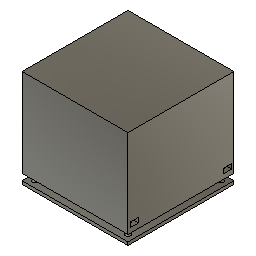
Indoors Test Enclosure (Autodesk Fusion 360 design; units mm, degrees)
Autodesk Fusion 360 part; units mm, degrees
note: some values were not read from the file. Set by a fixed rule: which sketch regions a step uses.
sketch "Sketch1" plane through (0, 0, 0) normal (0, 0, 1) x (1, 0, 0)
  line L0 (25.5, 25.5) -> (-25.5, 25.5)
  line L1 (-25.5, 25.5) -> (-25.5, -25.5)
  line L2 (-25.5, -25.5) -> (25.5, -25.5)
  line L3 (25.5, -25.5) -> (25.5, 25.5)
  line L4 (25.5, 25.5) -> (-25.5, -25.5) construction
  line L5 (-25.5, 25.5) -> (25.5, -25.5) construction
  circle A0 centre (0, 0) radius 22.6
  line L6 (-33, 33) -> (33, 33)
  line L7 (33, 33) -> (33, -33)
  line L8 (33, -33) -> (-33, -33)
  line L9 (-33, -33) -> (-33, 33)
  line L10 (-33, 33) -> (33, -33) construction
  line L11 (33, 33) -> (-33, -33) construction
  circle A1 centre (-29, 29) radius 1.6
  circle A2 centre (29, 29) radius 1.6
  circle A3 centre (-29, -29) radius 1.6
  circle A4 centre (29, -29) radius 1.6
  line L12 (-12.5, -12.5) -> (12.5, -12.5)
  line L13 (12.5, -12.5) -> (12.5, 12.5)
  line L14 (12.5, 12.5) -> (-12.5, 12.5)
  line L15 (-12.5, 12.5) -> (-12.5, -12.5)
  line L16 (-12.5, -12.5) -> (12.5, 12.5) construction
  line L17 (12.5, -12.5) -> (-12.5, 12.5) construction
  line L18 (-26, 29) -> (-27.5, 31.5981)
  line L19 (-27.5, 31.5981) -> (-30.5, 31.5981)
  line L20 (-30.5, 31.5981) -> (-32, 29)
  line L21 (-32, 29) -> (-30.5, 26.4019)
  line L22 (-30.5, 26.4019) -> (-27.5, 26.4019)
  line L23 (-27.5, 26.4019) -> (-26, 29)
  line L24 (30.5, 31.5981) -> (27.5, 31.5981)
  line L25 (32, 29) -> (30.5, 31.5981)
  line L26 (30.5, 26.4019) -> (32, 29)
  line L27 (27.5, 26.4019) -> (30.5, 26.4019)
  line L28 (26, 29) -> (27.5, 26.4019)
  line L29 (27.5, 31.5981) -> (26, 29)
  line L30 (-27.5, -26.4019) -> (-30.5, -26.4019)
  line L31 (-26, -29) -> (-27.5, -26.4019)
  line L32 (-27.5, -31.5981) -> (-26, -29)
  line L33 (-30.5, -31.5981) -> (-27.5, -31.5981)
  line L34 (-32, -29) -> (-30.5, -31.5981)
  line L35 (-30.5, -26.4019) -> (-32, -29)
  line L36 (30.5, -26.4019) -> (27.5, -26.4019)
  line L37 (32, -29) -> (30.5, -26.4019)
  line L38 (30.5, -31.5981) -> (32, -29)
  line L39 (27.5, -31.5981) -> (30.5, -31.5981)
  line L40 (26, -29) -> (27.5, -31.5981)
  line L41 (27.5, -26.4019) -> (26, -29)
  line L42 (-27.5, 31.5981) -> (-36.4083, 31.5981)
  line L43 (-36.4083, 31.5981) -> (-36.4083, 26.4019)
  line L44 (-36.4083, 26.4019) -> (-27.5, 26.4019)
  line L45 (-27.5, 26.4019) -> (-27.5, 31.5981)
  line L46 (-27.5, -26.4019) -> (-35.7888, -26.4019)
  line L47 (-35.7888, -26.4019) -> (-35.7888, -31.5981)
  line L48 (-35.7888, -31.5981) -> (-27.5, -31.5981)
  line L49 (-27.5, -31.5981) -> (-27.5, -26.4019)
  line L50 (27.5, 31.5981) -> (36.8588, 31.5981)
  line L51 (36.8588, 31.5981) -> (36.8588, 26.4019)
  line L52 (36.8588, 26.4019) -> (27.5, 26.4019)
  line L53 (27.5, 26.4019) -> (27.5, 31.5981)
  line L54 (27.5, -26.4019) -> (36.5392, -26.4019)
  line L55 (36.5392, -26.4019) -> (36.5392, -31.5981)
  line L56 (36.5392, -31.5981) -> (27.5, -31.5981)
  line L57 (27.5, -31.5981) -> (27.5, -26.4019)
  point P0 (29, 29)
  point P1 (-29, -29)
  point P2 (29, -29)
  point P3 (-29, 29)
  dimension "d1" = 51
  dimension "d2" = 51
  dimension "d3" = 45.2
  dimension "d4" = 66
  dimension "d5" = 66
  dimension "d6" = 3.2
  dimension "d9" = 58
  dimension "d10" = -58
  dimension "d13" = 58
  dimension "d14" = -58
  dimension "d23" = 25
  dimension "d24" = 25
  dimension "d28" = 3
  dimension "d31" = 58
  dimension "d32" = -58
  constraint horizontal L0
  constraint perpendicular L0 L1
  constraint parallel L0 L2
  constraint parallel L1 L3
  constraint coincident L4 A0.centre
  constraint coincident L5 A0.centre
  constraint coincident A0.centre origin
  constraint horizontal L6
  constraint perpendicular L6 L7
  constraint parallel L6 L8
  constraint parallel L7 L9
  constraint coincident L10 A0.centre
  constraint coincident L11 A0.centre
  constraint coincident L10 P3
  constraint horizontal L12
  constraint perpendicular L12 L13
  constraint parallel L12 L14
  constraint parallel L13 L15
  constraint coincident L16 A0.centre
  constraint coincident L17 A0.centre
  constraint coincident P3 A1.centre
  constraint horizontal L42
  constraint vertical L43
  constraint horizontal L44
  constraint vertical L45
  constraint horizontal L46
  constraint vertical L47
  constraint horizontal L48
  constraint vertical L49
  constraint horizontal L50
  constraint vertical L51
  constraint horizontal L52
  constraint vertical L53
  constraint horizontal L54
  constraint vertical L55
  constraint horizontal L56
  constraint vertical L57
  measures "d1" distance of L1.end L2.end
  measures "d2" distance of L0.end L1.end
  measures "d3" diameter of A0
  measures "d4" distance of L7.end L8.end
  measures "d5" distance of L6.end L7.end
  measures "d6" diameter of A1
  measures "d23" distance of L13.end L14.end
  measures "d24" distance of L12.end L13.end
  measures "d28" distance of L18.start P3
extrude "Extrude1" add sketch "Sketch1" along normal blind 55 contours L0 L1 L2 L3 | A0 | L6 L7 L8 L9 L18 L19 L22 L23 L24 L27 L28 L29 L30 L31 L32 L33 L36 L39 L40 L41 L42 L44 L46 L48 L50 L52 L54 L56 | L9 L20 L21 L42 L44 | L7 L25 L26 L50 L52 | A1 L19 L20 L21 L22 L42 L44 L45 | A2 L24 L25 L26 L27 L50 L52 L53 | L9 L34 L35 L46 L48 | A1 L18 L23 L45 | L7 L37 L38 L54 L56 | A2 L28 L29 L53 | A3 L30 L33 L34 L35 L46 L48 L49 | A1 L45 | A1 L45 | A4 L36 L37 L38 L39 L54 L56 L57 | A2 L53 | A2 L53 | A3 L31 L32 L49 | A4 L40 L41 L57 | A3 L49 | A3 L49 | A4 L57 | A4 L57 | L12 L13 L14 L15 makes body 1
extrude "Extrude2" cut sketch "Sketch1" along normal blind 52 contours A0 | L12 L13 L14 L15 bodies 1
extrude "Extrude3" cut sketch "Sketch1" along normal blind 2 contours L0 L1 L2 L3 bodies 1
extrude "Extrude4" cut sketch "Sketch1" along normal blind 10 contours A1 L45 | A1 L45 | A2 L53 | A2 L53 | A3 L49 | A3 L49 | A4 L57 | A4 L57 bodies 1
extrude "Extrude5" add sketch "Sketch1" against normal blind 1 from surface at -5 separate body contours L0 L1 L2 L3 | A0 | L6 L7 L8 L9 L18 L19 L22 L23 L24 L27 L28 L29 L30 L31 L32 L33 L36 L39 L40 L41 L42 L44 L46 L48 L50 L52 L54 L56 | L9 L20 L21 L42 L44 | L7 L25 L26 L50 L52 | A1 L19 L20 L21 L22 L42 L44 L45 | A2 L24 L25 L26 L27 L50 L52 L53 | L9 L34 L35 L46 L48 | A1 L18 L23 L45 | L7 L37 L38 L54 L56 | A2 L28 L29 L53 | A3 L30 L33 L34 L35 L46 L48 L49 | A4 L36 L37 L38 L39 L54 L56 L57 | A3 L31 L32 L49 | A4 L40 L41 L57 makes body 2
extrude "Extrude6" cut sketch "Sketch1" along normal blind 3 from surface at 3 contours L9 L20 L21 L42 L44 | L9 L42 L43 L44 | L7 L50 L51 L52 | L7 L25 L26 L50 L52 | A1 L19 L20 L21 L22 L42 L44 L45 | A2 L24 L25 L26 L27 L50 L52 L53 | L9 L34 L35 L46 L48 | L9 L46 L47 L48 | A1 L18 L23 L45 | L7 L37 L38 L54 L56 | A2 L28 L29 L53 | A3 L30 L33 L34 L35 L46 L48 L49 | A1 L45 | A1 L45 | A4 L36 L37 L38 L39 L54 L56 L57 | A2 L53 | A2 L53 | A3 L31 L32 L49 | A4 L40 L41 L57 | A3 L49 | A3 L49 | A4 L57 | A4 L57 bodies 1
extrude "Extrude7" add sketch "Sketch1" against normal blind 1 from surface at -4 contours L6 L7 L8 L9 L18 L19 L22 L23 L24 L27 L28 L29 L30 L31 L32 L33 L36 L39 L40 L41 L42 L44 L46 L48 L50 L52 L54 L56 | L9 L20 L21 L42 L44 | L7 L25 L26 L50 L52 | A1 L19 L20 L21 L22 L42 L44 L45 | A2 L24 L25 L26 L27 L50 L52 L53 | L9 L34 L35 L46 L48 | A1 L18 L23 L45 | L7 L37 L38 L54 L56 | A2 L28 L29 L53 | A3 L30 L33 L34 L35 L46 L48 L49 | A4 L36 L37 L38 L39 L54 L56 L57 | A3 L31 L32 L49 | A4 L40 L41 L57 bodies 2
